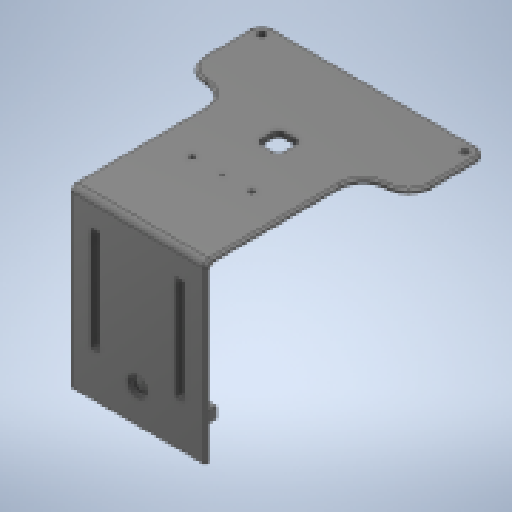
# Autodesk Inventor part: gripper_case_front
Saved by Autodesk Inventor 2026.2 (Build 302298010, 298A)
## iProperties
Created: 2026-05-24
Part Number: gripper_case_front
Material: ABS Plastic
Document SubType Name: Modeling
Designer: chris
Density: 1.06 g/cm^3
Appearance: Smooth - White
Author: chris
Autodesk Inventor part; units mm, degrees
ref_plane "YZ Plane" through (0, 0, 0) normal (1, 0, 0) x (0, 1, 0)
ref_plane "XZ Plane" through (0, 0, 0) normal (0, 1, 0) x (-1, 0, 0)
ref_plane "XY Plane" through (0, 0, 0) normal (0, 0, 1) x (1, 0, 0)
sketch "Sketch1" plane through (0, 0, 0) normal (0, 1, 0) x (-1, 0, 0)
  line L0 (60, 105) -> (-60, 105)
  line L1 (-60, 105) -> (-60, -105)
  line L2 (-60, -105) -> (60, -105)
  line L3 (60, -105) -> (60, 105)
  line L4 (60, 105) -> (-60, -105) construction
  line L5 (-60, 105) -> (60, -105) construction
  line L6 (100, -35) -> (-100, -35)
  line L7 (-100, -35) -> (-100, -105)
  line L8 (-100, -105) -> (100, -105)
  line L9 (100, -105) -> (100, -35)
  line L10 (100, -35) -> (-100, -105) construction
  line L11 (-100, -35) -> (100, -105) construction
  point P0 (0, 0)
  point P1 (0, -70)
  point P2 (-60, -35)
  point P3 (60, -35)
  dimension "d0" = 120
  dimension "d1" = 210
  dimension "d2" = 70
  dimension "d3" = 200
  constraints: 24 end point, 4 midpoint, 4 parallel, 2 horizontal, 2 perpendicular, 1 collinear, 1 vertical alignment
  measures "d0" distance of L2.end L1.end
  measures "d1" distance of L1.end L0.end
  measures "d2" distance of L6.end L7.end
  measures "d3" distance of L6.start L6.end
extrude "Extrusion1" add sketch "Sketch1" along normal blind 5
sketch "Sketch2" plane through (0, 5, 0) normal (0, 1, 0) x (1, 0, 0)
  circle A0 centre (-90, 95) radius 3.1
  circle A1 centre (90, 95) radius 3.1
  line L0 (100, 105) -> (-100, 105) projected
  line L1 (-100, 105) -> (-100, 35) projected
  line L2 (100, 35) -> (100, 105) projected
  point P0 (0, 0)
  dimension "d6" = 6.2
  dimension "d7" = 6.2
  dimension "d8" = 10
  dimension "d9" = 10
  dimension "d10" = 10
  constraints: 2 centre point, 1 horizontal alignment
  measures "d6" diameter of A0
  measures "d7" diameter of A1
  measures "d8" distance from line of L0 A0.centre
  measures "d9" distance from line of L1 A0.centre
  measures "d10" distance from line of L2 A1.centre
extrude "Extrusion2" cut sketch "Sketch2" against normal blind 5
sketch "Sketch3" plane through (0, 0, 0) normal (0, -1, 0) x (1, 0, 0)
  line L0 (-60, 105) -> (60, 105)
  line L1 (60, 105) -> (60, 100)
  line L2 (60, 100) -> (-60, 100)
  line L3 (-60, 100) -> (-60, 105)
  line L4 (-60, 105) -> (60, 100) construction
  line L5 (60, 105) -> (-60, 100) construction
  line L6 (60, 105) -> (60, -35) projected
  line L7 (-60, -35) -> (-60, 105) projected
  line L8 (-60, 105) -> (60, 105) projected
  point P0 (0, 0)
  point P1 (0, 102.5)
  dimension "d13" = 5
  constraints: 12 end point, 3 collinear, 2 midpoint, 2 parallel, 1 horizontal, 1 perpendicular
  measures "d13" distance of L2.end L0.start
extrude "Extrusion3" add sketch "Sketch3" along normal blind 150
fillet "Fillet1" radius 20 4 edges at (-60, 2.5, -35) (60, 2.5, -35) (100, 2.5, -35) (-100, 2.5, -35)
fillet "Fillet2" radius 10 2 edges at (100, 2.5, -105) (-100, 2.5, -105)
fillet "Fillet3" radius 5 2 edges at (0, 0, 100) (0, 5, 105)
fillet "Fillet4" radius 2 30 edges at (60, 3.5355, 103.5355) (60, 5, 42.4997) (80, 5, -35) (94.1423, 5, -40.8577) (100, 5, -74.9998) (97.0711, 5, -102.0711) (0, 5, -105) (-97.0711, 5, -102.0711) (-100, 5, -74.9997) (-94.1423, 5, -40.8577) (-80, 5, -35) (-60, 5, 42.4998) (-60, 3.5355, 103.5355) (-60, -75, 105) (60, -75, 105) (60, -1.4645, 98.5355) (60, 0, 39.9998) (80, 0, -35) (94.1423, 0, -40.8577) (100, 0, -74.9998) (97.0711, 0, -102.0711) (0, 0, -105) (-97.0711, 0, -102.0711) (-100, 0, -74.9997) (-94.1423, 0, -40.8577) (-80, 0, -35) (-60, 0, 39.9998) (-60, -1.4645, 98.5355) (-60, -77.5, 100) (60, -77.5, 100)
sketch "Sketch4" plane through (0, 5, 0) normal (0, 1, 0) x (1, 0, 0)
  point P0 (0, 0)
  point P1 (-26.5, -30)
  point P2 (26.5, -30)
  dimension "d20" = 26.5
  dimension "d21" = 30
  dimension "d23" = 26.5
  constraints: 1 horizontal alignment
  measures "d20" horizontal distance of point (-26.5, -30) point (0, 0)
  measures "d21" vertical distance of point (-26.5, -30) point (0, 0)
  measures "d23" horizontal distance of point (26.5, -30) point (0, 0)
hole "Hole1" at (-26.5, 5, 30) at (26.5, 5, 30) direction (0, -1, 0) diameter 4.2 end through all
sketch "Sketch6" plane through (0, 5, 0) normal (0, 1, 0) x (1, 0, 0)
  line L0 (-10, 30) -> (10, 30)
  line L1 (10, 30) -> (10, 10)
  line L2 (10, 10) -> (-10, 10)
  line L3 (-10, 10) -> (-10, 30)
  line L4 (-10, 30) -> (10, 10) construction
  line L5 (10, 30) -> (-10, 10) construction
  point P0 (0, 0)
  point P1 (0, 20)
  dimension "d37" = 20
  dimension "d38" = 20
  dimension "d39" = 20
  constraints: 12 end point, 2 midpoint, 2 parallel, 1 horizontal, 1 perpendicular, 1 vertical alignment
  measures "d37" distance of L0.end L1.end
  measures "d38" distance of L1.end L2.end
  measures "d39" distance of point (0, 20) point (0, 0)
extrude "Extrusion5" cut sketch "Sketch6" against normal blind 150
fillet "Fillet5" radius 5 4 edges at (-10, 2.5, -30) (10, 2.5, -30) (-10, 2.5, -10) (10, 2.5, -10)
sketch "Sketch7" plane through (-58, 0, 105) normal (0, 0, 1) x (1, 0, 0)
  line L0 (18, -20) -> (23, -20)
  line L1 (23, -20) -> (23, -110)
  line L2 (23, -110) -> (18, -110)
  line L3 (18, -110) -> (18, -20)
  line L4 (93, -20) -> (98, -20)
  line L5 (98, -20) -> (98, -110)
  line L6 (98, -110) -> (93, -110)
  line L7 (93, -110) -> (93, -20)
  line L8 (-2, 0) -> (-2, -150) projected
  line L9 (118, -150) -> (118, 0) projected
  line L10 (116, -150) -> (0, -150) projected
  point P0 (58, 0)
  dimension "d43" = 5
  dimension "d44" = 5
  dimension "d45" = 90
  dimension "d46" = 20
  dimension "d47" = 20
  dimension "d48" = 40
  constraints: 16 end point, 4 parallel, 2 horizontal, 2 perpendicular, 2 point on line
  measures "d43" distance of L1.end L2.end
  measures "d44" distance of L5.end L6.end
  measures "d45" distance of L0.end L1.end
  measures "d46" distance between parallel lines of L8 L3
  measures "d47" distance between parallel lines of L9 L5
  measures "d48" distance between parallel lines of L10 L2
extrude "Extrusion6" cut sketch "Sketch7" against normal blind 10
fillet "Fillet6" radius 1 8 edges at (40, -65, 105) (37.5, -20, 105) (35, -65, 105) (37.5, -110, 105) (-35, -65, 105) (-40, -65, 105) (-37.5, -110, 105) (-37.5, -20, 105)
sketch "Sketch8" plane through (-58, 0, 105) normal (0, 0, 1) x (1, 0, 0)
  circle A0 centre (58, -120) radius 7.5
  line L0 (116, -150) -> (0, -150) projected
  point P0 (58, 0)
  dimension "d52" = 15
  dimension "d53" = 30
  constraints: 1 centre point
  measures "d52" diameter of A0
  measures "d53" distance from line of L0 A0.centre
extrude "Extrusion7" cut sketch "Sketch8" against normal blind 10
sketch "Sketch11" plane through (58, -5, 100) normal (0, 0, -1) x (-1, 0, 0)
  line L0 (28, -135) -> (88, -135)
  line L1 (88, -135) -> (88, -145)
  line L2 (88, -145) -> (28, -145)
  line L3 (28, -145) -> (28, -135)
  line L4 (116, -145) -> (0, -145) projected
  point P0 (58, 5)
  point P1 (118, -145)
  dimension "d68" = 10
  dimension "d69" = 60
  dimension "d70" = 30
  constraints: 8 end point, 2 parallel, 1 collinear, 1 horizontal, 1 perpendicular
  measures "d68" distance of L2.end L0.start
  measures "d69" distance of L0.start L0.end
  measures "d70" distance from line of point (118, -145) L1
extrude "Extrusion9" add sketch "Sketch11" along normal blind 35
sketch "Sketch12" plane through (0, -150, 0) normal (0, -1, 0) x (1, 0, 0)
  circle A0 centre (-25, 70) radius 2.1
  circle A1 centre (25, 70) radius 2.1
  line L0 (30, 65) -> (-30, 65) projected
  line L1 (30, 100) -> (30, 65) projected
  line L2 (-30, 100) -> (-30, 65) projected
  point P0 (0, 0)
  dimension "d73" = 4.2
  dimension "d74" = 4.2
  dimension "d75" = 5
  dimension "d76" = 5
  dimension "d77" = 5
  dimension "d78" = 5
  constraints: 2 centre point
  measures "d73" diameter of A0
  measures "d74" diameter of A1
  measures "d75" distance from line of L0 A1.centre
  measures "d76" distance from line of L1 A1.centre
  measures "d77" distance from line of L2 A0.centre
  measures "d78" distance from line of L0 A0.centre
fillet "Fillet7" radius 1 1 edges at (-7.5, -120, 105)
extrude "Extrusion10" cut sketch "Sketch12" against normal blind 35
sketch "Sketch13" plane through (0, -150, 0) normal (0, -1, 0) x (1, 0, 0)
  circle A0 centre (25, 70) radius 2.1 projected
  circle A1 centre (-25, 70) radius 2.1 projected
  arc A2 (-60, 102) -> (-58, 100) centre (-58, 102) ccw projected
  line L0 (-58, 100) -> (-30, 100) projected
  line L1 (-30, 100) -> (-30, 65) projected
  line L2 (30, 65) -> (-30, 65) projected
  line L3 (30, 100) -> (30, 65) projected
  line L4 (30, 100) -> (58, 100) projected
  arc A3 (58, 100) -> (60, 102) centre (58, 102) ccw projected
  line L5 (60, 102) -> (60, 103) projected
  arc A4 (60, 103) -> (58, 105) centre (58, 103) ccw projected
  line L6 (58, 105) -> (-58, 105) projected
  arc A5 (-58, 105) -> (-60, 103) centre (-58, 103) ccw projected
  line L7 (-60, 103) -> (-60, 102) projected
  circle A6 centre (-25, 70) radius 4
  circle A7 centre (25, 70) radius 4
  point P0 (0, 0)
  dimension "d82" = 8
  dimension "d83" = 8
  constraints: 2 centre point, 2 coincident
  measures "d82" diameter of A6
  measures "d83" diameter of A7
extrude "Extrusion11" cut sketch "Sketch13" against normal blind 5 contours A6 | A7
sketch "Sketch14" plane through (0, 5, 0) normal (0, 1, 0) x (1, 0, 0)
  circle A0 centre (0, -30) radius 1
  circle A1 centre (-26.5, -30) radius 2.1 projected
  point P0 (0, 0)
  dimension "d86" = 2
  constraints: 1 centre point, 1 horizontal alignment
  measures "d86" diameter of A0
extrude "Extrusion12" cut sketch "Sketch14" against normal blind 10 contours A0
body "Solid1"
